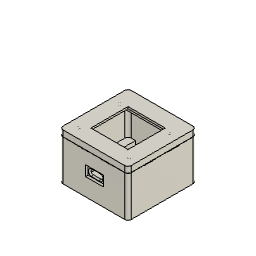
TinkerPod_v1_case (Autodesk Fusion 360 design; units mm, degrees)
Autodesk Fusion 360 part; units mm, degrees
sketch "Sketch1" plane through (0, 0, 0) normal (0, 0, 1) x (1, 0, 0)
  line L0 (0, 0) -> (44.5, 0)
  line L1 (44.5, 0) -> (44.5, 37)
  line L2 (44.5, 37) -> (0, 37)
  line L3 (0, 37) -> (0, 0)
  dimension "d1" = 44.5
  dimension "d2" = 37
  constraint horizontal L0
  constraint vertical L1
  constraint horizontal L2
  constraint vertical L3
  constraint coincident L0.start L3.end
  measures "d1" distance of L0.start L0.end
  measures "d2" distance of L0.start L2.end
extrude "Extrude1" add sketch "Sketch1" along normal blind 1.66 makes body 1 in component "Screen"
sketch "Sketch2" plane through (0, 0, 1.66) normal (0, 0, 1) x (-1, 0, 0)
  line L0 (0, -37) -> (0, 0)
  line L1 (0, 0) -> (-44.5, 0)
  line L2 (-44.5, 0) -> (-44.5, -37)
  line L3 (-44.5, -37) -> (0, -37)
  line L4 (-2.5, -34.5) -> (-42, -34.5)
  line L5 (-42, -34.5) -> (-42, -2.5)
  line L6 (-42, -2.5) -> (-2.5, -2.5)
  line L7 (-2.5, -2.5) -> (-2.5, -34.5)
  dimension "d5" = 2.5
  dimension "d6" = 2.5
  dimension "d7" = 2.5
  dimension "d8" = 2.5
  constraint horizontal L4
  constraint vertical L5
  constraint horizontal L6
  constraint vertical L7
  measures "d5" distance of L0 L7
  measures "d6" distance of L1 L6
  measures "d7" distance of L3 L4
  measures "d8" distance of L2 L5
hole "Hole1" at (2.5, 34.5, 1.66) at (42, 34.5, 1.66) at (42, 2.5, 1.66) at (2.5, 2.5, 1.66) direction (0, 0, -1) diameter 3 depth 5 tip angle 118 bodies 1 in component "Screen"
sketch "Sketch3" plane through (0, 0, 1.66) normal (0, 0, 1) x (1, 0, 0)
  line L0 (5.3, 37) -> (39.3, 37)
  line L1 (39.3, 37) -> (39.3, 0)
  line L2 (39.3, 0) -> (5.3, 0)
  line L3 (5.3, 0) -> (5.3, 37)
  line L4 (2.5, 2.5) -> (2.5, 34.5)
  line L5 (0, 0) -> (44.5, 0)
  line L6 (44.5, 37) -> (0, 37) construction
  line L7 (22.25, 37) -> (22.3, 0) construction
  line L8 (5.8, 36.8) -> (38.8, 36.8)
  line L9 (38.8, 36.8) -> (38.8, 3.8)
  line L10 (38.8, 3.8) -> (5.8, 3.8)
  line L11 (5.8, 3.8) -> (5.8, 36.8)
  line L12 (5.3, 20.2131) -> (5.8, 20.2131) construction
  line L13 (38.8, 20) -> (39.3, 20) construction
  dimension "d12" = 2.8
  dimension "d13" = 34
  dimension "d15" = 33
  dimension "d16" = 33
  dimension "d18" = 3.8
  constraint horizontal L0
  constraint vertical L1
  constraint horizontal L2
  constraint vertical L3
  constraint collinear L0 L6
  constraint collinear L2 L5
  constraint midpoint L6 L7.start
  constraint midpoint L2 L7.end
  constraint horizontal L8
  constraint vertical L9
  constraint horizontal L10
  constraint vertical L11
  constraint coincident L3 L12.start
  constraint coincident L11 L12.end
  constraint perpendicular L11 L12
  constraint coincident L9 L13.start
  constraint coincident L1 L13.end
  constraint perpendicular L1 L13
  constraint equal L12 L13
  measures "d12" distance of L3 L4
  measures "d13" distance of L1 L3
  measures "d15" distance of L8.start L8.end
  measures "d16" distance of L8.start L10.end
  measures "d18" distance of L2 L10
extrude "Extrude2" add sketch "Sketch3" along normal blind 1.44 bodies 1 in component "Screen"
extrude "Extrude3" add 1 faces at (27.8, 14.8, 1.66) along direction (0, 0, 1) blind 1.6 on bodies 1 bodies 1 in component "Screen"
sketch "ScreenBorders" plane through (0, 0, 3.26) normal (0, 0, 1) x (-1, 0, 0)
  line L0 (-22.3, -36.8) -> (-22.3, -3.8) construction
  line L1 (-5.8, -20.3) -> (-38.8, -20.3) construction
  line L2 (-7.8725, -35.8) -> (-36.7275, -35.8)
  line L3 (-36.7275, -35.8) -> (-36.7275, -6.945)
  line L4 (-36.7275, -6.945) -> (-7.8725, -6.945)
  line L5 (-7.8725, -6.945) -> (-7.8725, -35.8)
  line L6 (-5.8, -18.8419) -> (-7.8725, -18.8419) construction
  line L7 (-36.7275, -18.8419) -> (-38.8, -18.8419) construction
  line L8 (-35.7275, -7.945) -> (-8.8725, -7.945)
  line L9 (-8.8725, -7.945) -> (-8.8725, -34.8)
  line L10 (-8.8725, -34.8) -> (-35.7275, -34.8)
  line L11 (-35.7275, -34.8) -> (-35.7275, -7.945)
  line L12 (-38.8, -3.8) -> (-38.8, -36.8)
  line L13 (-38.8, -36.8) -> (-5.8, -36.8)
  line L14 (-5.8, -36.8) -> (-5.8, -3.8)
  line L15 (-5.8, -3.8) -> (-38.8, -3.8)
  dimension "d23" = 28.855
  dimension "d24" = 28.855
  dimension "d28" = 1
  constraint horizontal L2
  constraint vertical L3
  constraint horizontal L4
  constraint vertical L5
  constraint coincident L5 L6.end
  constraint perpendicular L5 L6
  constraint coincident L3 L7.start
  constraint equal L6 L7
  measures "d23" distance of L2.start L2.end
  measures "d24" distance of L2.start L4.end
fillet "Fillet1" radius 2 4 edges at (0, 0, 0.83) (44.5, 0, 0.83) (44.5, 37, 0.83) (0, 37, 0.83) on bodies 1 in component "Screen"
sketch "Sketch6" plane through (0, 0, 0) normal (0, 0, 1) x (1, 0, 0)
  line L0 (-1.95, 45.5725) -> (46.45, 45.5725)
  line L1 (46.45, 45.5725) -> (46.45, -2.8275)
  line L2 (46.45, -2.8275) -> (-1.95, -2.8275)
  line L3 (-1.95, -2.8275) -> (-1.95, 45.5725)
  line L4 (44.5, 37) -> (0, 37)
  line L5 (44.5, 0) -> (44.5, 37)
  line L6 (0, 37) -> (0, 0)
  line L7 (0, 0) -> (44.5, 0)
  line L8 (22.25, 85.4) -> (22.25, -2.8275) construction
  line L9 (0, 18.5) -> (-1.95, 18.5) construction
  line L10 (44.5, 18.5) -> (46.45, 18.5) construction
  line L11 (7.8725, 35.8) -> (36.7275, 35.8) construction
  line L12 (7.8725, 6.945) -> (7.8725, 35.8) construction
  line L13 (36.7275, 6.945) -> (7.8725, 6.945) construction
  line L14 (36.7275, 35.8) -> (36.7275, 6.945) construction
  line L15 (25, -2.8275) -> (25, 6.945) construction
  line L16 (25, 35.8) -> (25, 45.5725) construction
  dimension "d31" = 48.4
  dimension "d32" = 48.4
  constraint horizontal L0
  constraint vertical L1
  constraint horizontal L2
  constraint vertical L3
  constraint coincident L2 L8.end
  constraint midpoint L6 L9.start
  constraint coincident L3 L9.end
  constraint perpendicular L3 L9
  constraint midpoint L5 L10.start
  constraint coincident L1 L10.end
  constraint perpendicular L1 L10
  constraint equal L9 L10
  constraint coincident L2 L15.start
  constraint coincident L13 L15.end
  constraint perpendicular L13 L15
  constraint coincident L11 L16.start
  constraint coincident L0 L16.end
  constraint perpendicular L0 L16
  constraint equal L15 L16
  measures "d31" distance of L0.start L0.end
  measures "d32" distance of L0.start L2.end
extrude "Extrude1'" add sketch "Sketch6" along normal blind 3.26 and the other way blind 30 separate body contours L0 L1 L2 L3 | L4 L5 L6 L7 makes body 2 in component "Case"
shell "Shell1" thickness 1.5 outward yes removed faces 0 bodies 2 in component "Case"
extrude "Extrude2'" cut sketch "ScreenBorders" along normal blind 8 contours L2 L3 L4 L5 | L8 L9 L10 L11 bodies 2 in component "Case"
ref_plane "WorkPlane1" through (22.25, 21.3725, 3.26) normal (0, 0, -1) x (-1, 0, 0)
sketch "Sketch8" plane through (0, 0, 3.26) normal (0, 0, -1) x (-1, 0, 0)
  arc A0 (0, 35) -> (-2, 37) centre (-2, 35) ccw
  line L0 (-2, 37) -> (-42.5, 37)
  arc A1 (-42.5, 37) -> (-44.5, 35) centre (-42.5, 35) ccw
  line L1 (-44.5, 35) -> (-44.5, 2)
  arc A2 (-44.5, 2) -> (-42.5, 0) centre (-42.5, 2) ccw
  line L2 (-42.5, 0) -> (-2, 0)
  arc A3 (-2, 0) -> (0, 2) centre (-2, 2) ccw
  line L3 (0, 2) -> (0, 35)
  line L4 (-45.1, 35) -> (-45.1, 2)
  arc A4 (-45.1, 2) -> (-42.5, -0.6) centre (-42.5, 2) ccw
  line L5 (-42.5, -0.6) -> (-2, -0.6)
  arc A5 (-2, -0.6) -> (0.6, 2) centre (-2, 2) ccw
  line L6 (0.6, 2) -> (0.6, 35)
  arc A6 (0.6, 35) -> (-2, 37.6) centre (-2, 35) ccw
  line L7 (-2, 37.6) -> (-42.5, 37.6)
  arc A7 (-42.5, 37.6) -> (-45.1, 35) centre (-42.5, 35) ccw
  line L8 (-47.95, -4.3275) -> (3.45, -4.3275)
  line L9 (3.45, -4.3275) -> (3.45, 47.0725)
  line L10 (3.45, 47.0725) -> (-47.95, 47.0725)
  line L11 (-47.95, 47.0725) -> (-47.95, -4.3275)
  line L12 (-5.3, 0) -> (-39.3, 0)
  line L13 (-39.3, 0) -> (-39.3, 37)
  line L14 (-39.3, 37) -> (-5.3, 37)
  line L15 (-5.3, 37) -> (-5.3, 0)
  line L16 (-39.9, -0.6) -> (-39.9, 37.6)
  line L17 (-39.9, 37.6) -> (-4.7, 37.6)
  line L18 (-4.7, 37.6) -> (-4.7, -0.6)
  line L19 (-4.7, -0.6) -> (-39.9, -0.6)
  line L20 (-7.8725, 35.8) -> (-7.8725, 6.945)
  line L21 (-7.8725, 6.945) -> (-36.7275, 6.945)
  line L22 (-36.7275, 6.945) -> (-36.7275, 35.8)
  line L23 (-36.7275, 35.8) -> (-7.8725, 35.8)
  line L24 (-46.45, -2.8275) -> (1.95, -2.8275)
  line L25 (1.95, -2.8275) -> (1.95, 45.5725)
  line L26 (1.95, 45.5725) -> (-46.45, 45.5725)
  line L27 (-46.45, 45.5725) -> (-46.45, -2.8275)
  dimension "d43" = 0.6
  dimension "d44" = -0.6
extrude "Extrude3'" add sketch "Sketch8" along normal blind 1.5 contours A0 L0 L2 A3 L3 L18 | A0 L0 L2 A3 L3 L5 A5 L6 A6 L7 L18 | L0 A1 L1 A2 L2 L4 A4 L5 L7 A7 L16 | L0 A1 L1 A2 L2 L16 bodies 2 in component "Case"
extrude "Extrude4" add sketch "Sketch8" along normal up to surface (3.26 mm away) contours L24 L25 L26 L27 bodies 2 in component "Case"
ref_plane "WorkPlane2" through (0, 0, 0) normal (0, 1, 0) x (0, 0, 1)
sketch "Measurements" plane through (0, 0, 0) normal (0, 1, 0) x (1, 0, 0)
  line L0 (-3.45, 31.5) -> (-3.45, -4.76)
  line L1 (-3.45, -4.76) -> (47.95, -4.76)
  line L2 (47.95, -4.76) -> (47.95, 31.5)
  line L3 (47.95, 31.5) -> (-3.45, 31.5)
  line L4 (2, 0) -> (2, -1.66)
  line L5 (2, -1.66) -> (5.3, -1.66)
  line L6 (5.3, -1.66) -> (5.3, -3.1)
  line L7 (5.3, -3.1) -> (39.3, -3.1)
  line L8 (39.3, -3.1) -> (39.3, -1.66)
  line L9 (39.3, -1.66) -> (42.5, -1.66)
  line L10 (42.5, -1.66) -> (42.5, 0)
  line L11 (42.5, 0) -> (2, 0)
  line L12 (44.5, -1.66) -> (42.5, -1.66)
  line L13 (44.5, -1.66) -> (44.5, 0)
  line L14 (42.5, 0) -> (44.5, 0)
  line L15 (42.5, 0) -> (42.5, -1.66)
  line L16 (40.5, 0) -> (43.5, 0)
  line L17 (43.5, -1.66) -> (40.5, -1.66)
  line L18 (36.7275, -3.26) -> (7.8725, -3.26)
hole "Hole1'" at (42, 34.5, 1.66) at (42, 2.5, 1.66) at (2.5, 34.5, 1.66) at (2.5, 2.5, 1.66) direction (0, 0, 1) diameter 2.4 depth 2.5 tip angle 180 bodies 2 in component "Case"
ref_plane "WorkPlane3" through (22.25, 21.3725, -29) normal (0, 0, 1) x (1, 0, 0)
sketch "Sketch11" plane through (0, 0, -29) normal (0, 0, 1) x (1, 0, 0)
  line L0 (-1.95, -2.8275) -> (46.45, -2.8275)
  line L1 (46.45, -2.8275) -> (46.45, 45.5725)
  line L2 (46.45, 45.5725) -> (-1.95, 45.5725)
  line L3 (-1.95, 45.5725) -> (-1.95, -2.8275)
  line L4 (22.25, 45.5725) -> (22.25, -2.8275) construction
  line L5 (-1.95, 21.3725) -> (46.45, 21.3725) construction
  line L6 (4.25, 45.3725) -> (40.25, 45.3725)
  line L7 (40.25, 45.3725) -> (40.25, -2.6275)
  line L8 (40.25, -2.6275) -> (4.25, -2.6275)
  line L9 (4.25, -2.6275) -> (4.25, 45.3725)
  line L10 (25, 45.3725) -> (25, 45.5725) construction
  line L11 (40.25, 23) -> (46.45, 23) construction
  line L12 (4.25, 23) -> (-1.95, 23) construction
  line L13 (25, -2.6275) -> (25, -2.8275) construction
  dimension "d55" = 36
  dimension "d56" = 48
  constraint midpoint L2 L4.start
  constraint midpoint L0 L4.end
  constraint midpoint L3 L5.start
  constraint midpoint L1 L5.end
  constraint horizontal L6
  constraint vertical L7
  constraint horizontal L8
  constraint vertical L9
  constraint coincident L6 L10.start
  constraint coincident L2 L10.end
  constraint perpendicular L2 L10
  constraint coincident L7 L11.start
  constraint coincident L1 L11.end
  constraint perpendicular L1 L11
  constraint coincident L9 L12.start
  constraint coincident L3 L12.end
  constraint perpendicular L3 L12
  constraint equal L11 L12
  constraint coincident L8 L13.start
  constraint coincident L0 L13.end
  constraint perpendicular L0 L13
  constraint equal L10 L13
  measures "d55" distance of L6.start L6.end
  measures "d56" distance of L6.start L8.end
extrude "Extrude1''" add sketch "Sketch11" along normal blind 10 separate body contours L6 L7 L8 L9 makes body 3 in component "Controller"
sketch "Sketch12" plane through (0, 0, -19) normal (0, 0, 1) x (-1, 0, 0)
  line L0 (-4.25, 2.6275) -> (-40.25, 2.6275)
  line L1 (-40.25, 2.6275) -> (-40.25, -45.3725)
  line L2 (-40.25, -45.3725) -> (-4.25, -45.3725)
  line L3 (-4.25, -45.3725) -> (-4.25, 2.6275)
  line L4 (-38.25, 0.6275) -> (-38.25, -43.3725)
  line L5 (-38.25, -43.3725) -> (-6.25, -43.3725)
  line L6 (-6.25, -43.3725) -> (-6.25, 0.6275)
  line L7 (-6.25, 0.6275) -> (-38.25, 0.6275)
  dimension "d60" = -2
extrude "Extrude2''" add sketch "Sketch12" along normal blind 10 contours L4 L5 L6 L7 bodies 3 in component "Controller"
sketch "Sketch13" plane through (0, 0, -30) normal (0, 0, 1) x (-1, 0, 0)
  line L0 (1.95, 2.8275) -> (-46.45, 2.8275)
  line L1 (-46.45, 2.8275) -> (-46.45, -45.5725)
  line L2 (-46.45, -45.5725) -> (1.95, -45.5725)
  line L3 (1.95, -45.5725) -> (1.95, 2.8275)
  line L4 (-4.25, 2.6275) -> (-40.25, 2.6275)
  line L5 (-40.25, 2.6275) -> (-40.25, -45.3725)
  line L6 (-40.25, -45.3725) -> (-4.25, -45.3725)
  line L7 (-4.25, -45.3725) -> (-4.25, 2.6275)
  line L8 (-40.65, 3.0275) -> (-40.65, -45.7725)
  line L9 (-40.65, -45.7725) -> (-3.85, -45.7725)
  line L10 (-3.85, -45.7725) -> (-3.85, 3.0275)
  line L11 (-3.85, 3.0275) -> (-40.65, 3.0275)
  dimension "d63" = 0.4
extrude "Extrude5" add sketch "Sketch13" along normal blind 5 contours L0 L2 L3 L10 | L0 L1 L2 L8 bodies 2 in component "Case"
extrude "Extrude6" add 1 faces at (28.3833, 13.3058, -30) along direction (0, 0, 1) blind 0.8 on bodies 2 bodies 2 in component "Case"
sketch "USB C" plane through (0, -0.6275, 0) normal (0, -1, 0) x (1, 0, 0)
  line L0 (6.25, -19) -> (38.25, -19)
  line L1 (38.25, -19) -> (38.25, -9)
  line L2 (38.25, -9) -> (6.25, -9)
  line L3 (6.25, -9) -> (6.25, -19)
  line L4 (22.25, -9) -> (22.25, -19) construction
  line L5 (6.25, -14) -> (38.25, -14) construction
  line L6 (19.75, -15.6) -> (25.75, -15.6)
  arc A0 (25.75, -15.6) -> (25.75, -12.2) centre (25.75, -13.9) ccw
  line L7 (25.75, -12.2) -> (19.75, -12.2)
  arc A1 (19.75, -12.2) -> (19.75, -15.6) centre (19.75, -13.9) ccw
  dimension "d68" = 3.4
  dimension "d69" = 3.4
  dimension "d73" = 6
  dimension "d120" = 12.5
  constraint midpoint L2 L4.start
  constraint midpoint L0 L4.end
  constraint midpoint L3 L5.start
  constraint midpoint L1 L5.end
  constraint tangent L6 A0
  constraint tangent A0 L7
  constraint parallel L6 L7
  constraint tangent L7 A1
  constraint tangent L6 A1
  measures "d68" diameter of A0
  measures "d69" distance of L0 L6
  measures "d73" distance of A1.centre A0.centre
  measures "d120" distance of L1 A0.centre
ref_plane "WorkPlane4" through (22.25, 21.3725, -1.24) normal (0, 0, 1) x (1, 0, 0)
split "Split1" by plane through (22.25, 21.3725, -1.24) normal (0, 0, 1) bodies 2 makes body 4 at (0.3242, 26.1817, 4.76) in component "Case"
ref_plane "WorkPlane5" through (22.25, 21.3725, -31.5) normal (0, 0, -1) x (-1, 0, 0)
sketch "Sketch15" plane through (0, 0, -31.5) normal (0, 0, -1) x (-1, 0, 0)
  line L0 (-47.95, -4.3275) -> (3.45, -4.3275)
  line L1 (3.45, -4.3275) -> (3.45, 47.0725)
  line L2 (3.45, 47.0725) -> (-47.95, 47.0725)
  line L3 (-47.95, 47.0725) -> (-47.95, -4.3275)
  line L4 (-48.75, 47.8725) -> (-48.75, -5.1275)
  line L5 (-48.75, -5.1275) -> (4.25, -5.1275)
  line L6 (4.25, -5.1275) -> (4.25, 47.8725)
  line L7 (4.25, 47.8725) -> (-48.75, 47.8725)
  dimension "d79" = 0.8
extrude "Extrude7" add sketch "Sketch15" against normal blind 31.5 bodies 2 in component "Case"
ref_plane "WorkPlane6" through (22.25, 21.3725, 4.76) normal (0, 0, 1) x (1, 0, 0)
sketch "Sketch16" plane through (0, 0, 4.76) normal (0, 0, 1) x (1, 0, 0)
  line L0 (-3.45, -4.3275) -> (47.95, -4.3275)
  line L1 (47.95, -4.3275) -> (47.95, 47.0725)
  line L2 (47.95, 47.0725) -> (-3.45, 47.0725)
  line L3 (-3.45, 47.0725) -> (-3.45, -4.3275)
  line L4 (48.75, -5.1275) -> (48.75, 47.8725)
  line L5 (48.75, 47.8725) -> (-4.25, 47.8725)
  line L6 (-4.25, 47.8725) -> (-4.25, -5.1275)
  line L7 (-4.25, -5.1275) -> (48.75, -5.1275)
  dimension "d83" = 0.8
extrude "Extrude8" add sketch "Sketch16" against normal blind 4.6 bodies 4 in component "Case"
move_face "OffsetFaces1" offset -0.2 4 faces at (47.95, 29.9392, -0.7733) (30.8167, -4.3275, -0.3067) (13.6833, 47.0725, -0.7733) (-3.45, 12.8058, -0.7733) on bodies 4 in component "Case"
copy_body "Body->Comp1" bodies 4 removing the originals makes body 5 in component "Top"
copy_body "Body->Comp2" bodies 2 removing the originals makes body 6 in component "Bottom"
fillet "Fillet1'" radius 2.5 4 edges at (48.75, -5.1275, 2.46) (48.75, 47.8725, 2.46) (-4.25, 47.8725, 2.46) (-4.25, -5.1275, 2.46) on bodies 5 in component "Top"
fillet "Fillet1'" radius 2.5 4 edges at (-3.25, -4.1275, -0.54) (-3.25, 46.8725, -0.54) (47.75, -4.1275, -0.54) (47.75, 46.8725, -0.54) on bodies 5 in component "Top"
fillet "Fillet1'" radius 2.5 4 edges at (-1.95, 45.5725, -0.62) (-1.95, -2.8275, -0.62) (46.45, -2.8275, -0.62) (46.45, 45.5725, -0.62) on bodies 5 in component "Top"
fillet "Fillet1''" radius 2.5 4 edges at (-1.95, 45.5725, -13.12) (-1.95, -2.8275, -13.12) (46.45, -2.8275, -13.12) (46.45, 45.5725, -13.12) on bodies 6 in component "Bottom"
fillet "Fillet1''" radius 2.5 4 edges at (-3.45, 47.0725, -0.62) (-3.45, -4.3275, -0.62) (47.95, -4.3275, -0.62) (47.95, 47.0725, -0.62) on bodies 6 in component "Bottom"
fillet "Fillet1''" radius 2.5 4 edges at (48.75, -5.1275, -15.75) (48.75, 47.8725, -15.75) (-4.25, 47.8725, -15.75) (-4.25, -5.1275, -15.75) on bodies 6 in component "Bottom"
sketch "Sketch17" plane through (0, -5.1275, 0) normal (0, -1, 0) x (1, 0, 0)
  line L0 (-1.75, 0) -> (-1.75, -31.5)
  line L1 (-1.75, -31.5) -> (46.25, -31.5)
  line L2 (46.25, -31.5) -> (46.25, 0)
  line L3 (46.25, 0) -> (-1.75, 0)
  line L4 (25.75, -12.2) -> (19.75, -12.2)
  arc A0 (19.75, -12.2) -> (19.75, -15.6) centre (19.75, -13.9) ccw
  line L5 (19.75, -15.6) -> (25.75, -15.6)
  arc A1 (25.75, -15.6) -> (25.75, -12.2) centre (25.75, -13.9) ccw
extrude "Extrude1'''" cut sketch "Sketch17" against normal up to surface (2.3 mm away) contours L4 A0 L5 A1 bodies 6 in component "Bottom"
sketch "Sketch18" plane through (0, -5.1275, 0) normal (0, -1, 0) x (1, 0, 0)
  line L0 (25.75, -15.6) -> (19.75, -15.6)
  arc A0 (19.75, -12.2) -> (19.75, -15.6) centre (19.75, -13.9) ccw
  line L1 (19.75, -12.2) -> (25.75, -12.2)
  arc A1 (25.75, -15.6) -> (25.75, -12.2) centre (25.75, -13.9) ccw
  line L2 (-1.75, 0) -> (-1.75, -31.5)
  line L3 (-1.75, -31.5) -> (46.25, -31.5)
  line L4 (46.25, -31.5) -> (46.25, 0)
  line L5 (46.25, 0) -> (-1.75, 0)
  arc A2 (25.75, -15.6) -> (25.75, -12.2) centre (25.75, -13.9) ccw
  line L6 (25.75, -12.2) -> (19.75, -12.2)
  arc A3 (19.75, -12.2) -> (19.75, -15.6) centre (19.75, -13.9) ccw
  line L7 (19.75, -15.6) -> (25.75, -15.6)
  line L8 (16.75, -10.9) -> (28.75, -10.9)
  line L9 (28.75, -10.9) -> (28.75, -16.9)
  line L10 (28.75, -16.9) -> (16.75, -16.9)
  line L11 (16.75, -16.9) -> (16.75, -10.9)
  line L12 (16.75, -13.9) -> (18.05, -13.9) construction
  line L13 (27.45, -13.9) -> (28.75, -13.9) construction
  line L14 (22.75, -10.9) -> (22.75, -12.2) construction
  line L15 (22.75, -16.9) -> (22.75, -15.6) construction
  point P0 (19.75, -12.2)
  point P1 (19.75, -13.9)
  point P2 (19.75, -15.6)
  point P3 (25.75, -12.2)
  point P4 (25.75, -13.9)
  point P5 (25.75, -15.6)
  dimension "d101" = 12
  dimension "d102" = 6
  constraint horizontal L8
  constraint vertical L9
  constraint horizontal L10
  constraint vertical L11
  constraint midpoint L11 L12.start
  constraint midpoint A3 L12.end
  constraint midpoint A1 L13.start
  constraint midpoint L9 L13.end
  constraint perpendicular L11 L13
  constraint equal L12 L13
  constraint midpoint L8 L14.start
  constraint midpoint L6 L14.end
  constraint midpoint L10 L15.start
  constraint midpoint L7 L15.end
  measures "d101" distance of L8.start L8.end
  measures "d102" distance of L8.start L10.end
extrude "Extrude2'''" cut sketch "Sketch18" against normal blind 1 contours L8 L9 L10 L11 bodies 6 in component "Bottom"
fillet "Fillet4" radius 1 8 edges at (22.75, -4.1275, -15.6) (27.45, -4.1275, -13.9) (22.75, -4.1275, -12.2) (18.05, -4.1275, -13.9) (22.75, -2.8275, -15.6) (27.45, -2.8275, -13.9) (22.75, -2.8275, -12.2) (18.05, -2.8275, -13.9) on bodies 6 in component "Bottom"
chamfer "Chamfer1" distance 1 angle 45 4 edges at (22.75, -5.1275, -10.9) (16.75, -5.1275, -13.9) (28.75, -5.1275, -13.9) (22.75, -5.1275, -16.9) measured on face at (4.4167, -5.1275, -16.1333) measured on face at (4.4167, -5.1275, -16.1333) measured on face at (4.4167, -5.1275, -16.1333) measured on face at (4.4167, -5.1275, -16.1333) on bodies 6 in component "Bottom"
move_face "OffsetFaces1'" offset -0.1 1 faces at (-2.8167, 28.6058, -1.24) on bodies 5 in component "Top"
move_face "OffsetFaces1''" offset -0.1 1 faces at (47.45, 14.1392, -1.24) on bodies 6 in component "Bottom"
sketch "Sketch19" plane through (47.75, 0, 0) normal (1, 0, 0) x (0, 1, 0)
  line L0 (44.3725, -1.14) -> (44.3725, 0.16)
  line L1 (44.3725, 0.16) -> (-1.6275, 0.16)
  line L2 (-1.6275, 0.16) -> (-1.6275, -1.14)
  line L3 (-1.6275, -1.14) -> (44.3725, -1.14)
  line L4 (-1.6275, -0.49) -> (44.3725, -0.49) construction
  line L5 (7.5725, -0.29) -> (16.7725, -0.29)
  line L6 (16.7725, -0.29) -> (16.7725, -1.09)
  line L7 (16.7725, -1.09) -> (7.5725, -1.09)
  line L8 (7.5725, -1.09) -> (7.5725, -0.29)
  line L9 (35.1725, -1.09) -> (25.9725, -1.09)
  line L10 (25.9725, -0.29) -> (35.1725, -0.29)
  line L11 (25.9725, -1.09) -> (25.9725, -0.29)
  line L12 (35.1725, -0.29) -> (35.1725, -1.09)
  dimension "d121" = 9.2
  dimension "d122" = 0.8
  dimension "d123" = 0.2
  dimension "d124" = 9.2
  dimension "d127" = 18.4
  dimension "d128" = 0
  constraint midpoint L2 L4.start
  constraint midpoint L0 L4.end
  constraint horizontal L5
  constraint vertical L6
  constraint horizontal L7
  constraint vertical L8
  measures "d121" distance of L5.start L5.end
  measures "d122" distance of L5.start L7.end
  measures "d123" distance of L4 L5
  measures "d124" distance of L2 L8
extrude "Extrude1''''" add sketch "Sketch19" along normal blind 1 draft -45 contours L5 L6 L7 L8 | L9 L10 L11 L12 bodies 5 in component "Top"
sketch "Sketch20" plane through (0, 0, 4.76) normal (0, 0, 1) x (-1, 0, 0)
  arc A0 (4.25, 2.6275) -> (1.75, 5.1275) centre (1.75, 2.6275) ccw
  line L0 (1.75, 5.1275) -> (-46.25, 5.1275)
  arc A1 (-46.25, 5.1275) -> (-48.75, 2.6275) centre (-46.25, 2.6275) ccw
  line L1 (-48.75, 2.6275) -> (-48.75, -45.3725)
  arc A2 (-48.75, -45.3725) -> (-46.25, -47.8725) centre (-46.25, -45.3725) ccw
  line L2 (-46.25, -47.8725) -> (1.75, -47.8725)
  arc A3 (1.75, -47.8725) -> (4.25, -45.3725) centre (1.75, -45.3725) ccw
  line L3 (4.25, -45.3725) -> (4.25, 2.6275)
  line L4 (-7.8725, -6.945) -> (-7.8725, -35.8)
  line L5 (-7.8725, -35.8) -> (-36.7275, -35.8)
  line L6 (-36.7275, -35.8) -> (-36.7275, -6.945)
  line L7 (-36.7275, -6.945) -> (-7.8725, -6.945)
  line L8 (-36.7275, -6.945) -> (-7.8725, -35.8) construction
  line L9 (-36.7275, -35.8) -> (-7.8725, -6.945) construction
  point P0 (-22.3, -21.3725)
  constraint coincident L6.end L7.start
  constraint coincident L4.end L5.start
  constraint coincident L5.end L6.start
  constraint coincident L4.start L7.end
  constraint midpoint L9 P0
pattern_circular "C-Pattern1" count 4 over 360 about axis through (22.3, 21.3725, -48.24) along (0, 0, 1) of "Extrude1''''" in component "Top"
sketch "Sketch21" plane through (47.95, 0, 0) normal (-1, 0, 0) x (0, -1, 0)
  line L0 (-44.5725, 0) -> (-44.5725, -1.34)
  line L1 (-44.5725, -1.34) -> (1.8275, -1.34)
  line L2 (1.8275, -1.34) -> (1.8275, 0)
  line L3 (1.8275, 0) -> (-44.5725, 0)
  line L4 (-25.9725, -0.29) -> (-35.1725, -0.29)
  line L5 (-35.1725, -1.09) -> (-25.9725, -1.09)
  line L6 (-35.1725, -0.29) -> (-35.1725, -1.09)
  line L7 (-25.9725, -1.09) -> (-25.9725, -0.29)
  line L8 (-16.7725, -0.29) -> (-16.7725, -1.09)
  line L9 (-7.5725, -0.29) -> (-16.7725, -0.29)
  line L10 (-16.7725, -1.09) -> (-7.5725, -1.09)
  line L11 (-7.5725, -1.09) -> (-7.5725, -0.29)
extrude "Extrude3''" cut sketch "Sketch21" against normal blind 1 draft -45 contours L4 L5 L6 L7 | L8 L9 L10 L11 bodies 6 in component "Bottom"
pattern_circular "C-Pattern1'" count 4 over 360 about axis through (22.3, 21.3725, -48.24) along (0, 0, 1) of "Extrude3''" in component "Bottom"
component "Screen" placed x (1, 0, 0) y (0, 1, 0) z (0, 0, 1) at (0, 0, 0)
component "Case" placed x (1, 0, 0) y (0, 1, 0) z (0, 0, 1) at (0, 0, 0)
component "Controller" placed x (1, 0, 0) y (0, 1, 0) z (0, 0, 1) at (0, 0, 0)
component "Top" placed x (1, 0, 0) y (0, 1, 0) z (0, 0, 1) at (0, 0, 0) in component "Case"
component "Bottom" placed x (1, 0, 0) y (0, 1, 0) z (0, 0, 1) at (0, 0, 0) in component "Case"
equation "d34 = 1.60 mm + 1.66 mm"
equation "d123 = ( d122 / 2 ) - 0.2 mm"
